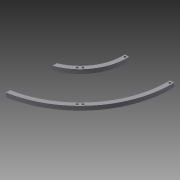
# Autodesk Inventor part: Upper Rails
Saved by Autodesk Inventor 2013 (Build 170138000, 138)
## iProperties
Created: 2013-01-26
Part Number: Upper Rails
Material: Generic
Document SubType Name: Modeling
Designer: actoennies
Density: 1 g/cm^3
Mass: 88.8713 g
Surface Area: 306.982 cm^2
Volume: 88.8713 cm^3
Author: actoennies
Autodesk Inventor part; units mm, degrees
ref_plane "YZ Plane" through (0, 0, 0) normal (1, 0, 0) x (0, 1, 0)
ref_plane "XZ Plane" through (0, 0, 0) normal (0, 1, 0) x (-1, 0, 0)
ref_plane "XY Plane" through (0, 0, 0) normal (0, 0, 1) x (1, 0, 0)
sketch "Sketch1" plane through (0, 0, 0) normal (0, 1, 0) x (-1, 0, 0)
  circle A0 centre (-193.0245, 202.0047) radius 4.7625
  circle A1 centre (-279.4, 0) radius 4.7625
  circle A2 centre (-202.0047, 193.0245) radius 4.7625
  arc A3 (-50.8, 268.2828) -> (-273.05, 0) centre (0, 0) ccw
  arc A4 (-50.8, 281.1982) -> (-285.75, 0) centre (0, 0) ccw
  line L0 (-285.75, 0) -> (-285.75, -6.35)
  line L1 (-285.75, -6.35) -> (-273.05, -6.35)
  line L2 (-273.05, -6.35) -> (-273.05, 0)
  circle A5 centre (-94.1906, 103.1708) radius 4.7625
  circle A6 centre (-139.7, 0) radius 4.7625
  circle A7 centre (-103.1708, 94.1906) radius 4.7625
  arc A8 (-50.8, 136.9305) -> (-146.05, 0) centre (0, 0) ccw
  line L3 (-146.05, 0) -> (-146.05, -6.35)
  line L4 (-146.05, -6.35) -> (-133.35, -6.35)
  line L5 (-133.35, -6.35) -> (-133.35, 0)
  arc A9 (-50.8, 123.2947) -> (-133.35, 0) centre (0, 0) ccw
  line L6 (-50.8, 123.2947) -> (-50.8, 136.9305)
  line L7 (-50.8, 268.2828) -> (-50.8, 281.1982)
  constraints: 16 end point, 10 centre point, 8 point on circle, 4 vertical, 2 horizontal, 33 other
extrude "Extrusion1" add sketch "Sketch1" along normal blind 12.7
sketch "Sketch2" plane through (0, 0, 0) normal (0, -1, 0) x (1, 0, 0)
  circle A0 centre (202.0047, 193.0245) radius 4.7625 projected
  circle A1 centre (193.0245, 202.0047) radius 4.7625 projected
  circle A2 centre (279.4, 0) radius 4.7625 projected
  arc A3 (133.35, 0) -> (50.8, 123.2947) centre (0, 0) ccw projected
  circle A4 centre (103.1708, 94.1906) radius 4.7625 projected
  circle A5 centre (94.1906, 103.1708) radius 4.7625 projected
  circle A6 centre (139.7, 0) radius 4.7625 projected
  arc A7 (146.05, 0) -> (50.8, 136.9305) centre (0, 0) ccw projected
  line L0 (50.8, 136.9305) -> (50.8, 123.2947) projected
  arc A8 (133.35, 0) -> (50.8, 123.2947) centre (0, 0) ccw projected
  line L1 (133.35, 0) -> (133.35, -6.35) projected
  line L2 (133.35, -6.35) -> (146.05, -6.35) projected
  line L3 (146.05, -6.35) -> (146.05, 0) projected
  circle A9 centre (202.0047, 193.0245) radius 3.3782
  circle A10 centre (193.0245, 202.0047) radius 3.3782
  circle A11 centre (279.4, 0) radius 3.3782
  circle A12 centre (139.7, 0) radius 3.3782
  circle A13 centre (94.1906, 103.1708) radius 3.3782
  circle A14 centre (103.1708, 94.1906) radius 3.3782
  dimension "d3" = 6.7564
  dimension "d4" = 6.7564
  dimension "d5" = 6.7564
  dimension "d6" = 6.7564
  dimension "d7" = 6.7564
  dimension "d8" = 6.7564
  constraints: 6 centre point, 6 coincident
  measures "d3" diameter of A9
  measures "d4" diameter of A10
  measures "d5" diameter of A11
  measures "d6" diameter of A12
  measures "d7" diameter of A13
  measures "d8" diameter of A14
extrude "Extrusion2" add sketch "Sketch2" against normal blind 12.7 contours A0 | A1 | A2 | A4 | A5 | A6
body "Solid1"
